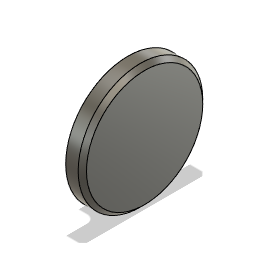
Button Cover Blank v1 (Autodesk Fusion 360 design; units mm, degrees)
Autodesk Fusion 360 part; units mm, degrees
sketch "Sketch1" plane through (0, 0, 0) normal (1, 0, 0) x (0, 0, -1)
  circle A0 centre (0, 0) radius 4
  line L0 (2, 2) -> (-2, 2)
  line L1 (-2, 2) -> (-2, -2)
  line L2 (-2, -2) -> (2, -2)
  line L3 (2, -2) -> (2, 2)
  line L4 (2, 2) -> (-2, -2) construction
  line L5 (-2, 2) -> (2, -2) construction
  dimension "d1" = 8
  dimension "d2" = 4
  dimension "d3" = 4
  constraint coincident A0.centre origin
  constraint horizontal L0
  constraint perpendicular L0 L1
  constraint parallel L0 L2
  constraint parallel L1 L3
  constraint coincident L4 A0.centre
  constraint coincident L5 A0.centre
  measures "d1" diameter of A0
  measures "d2" distance of L0.start L0.end
  measures "d3" distance of L0.start L2.end
extrude "Extrude1" add sketch "Sketch1" along normal blind 2
sketch "Sketch2" plane through (2, 0, 0) normal (1, 0, 0) x (0, 0, -1)
  line L0 (2, 2) -> (2, -2)
  line L1 (2, -2) -> (-2, -2)
  line L2 (-2, -2) -> (-2, 2)
  line L3 (-2, 2) -> (2, 2)
  circle A0 centre (0, 0) radius 4
  circle A1 centre (0, 0) radius 7.5
  dimension "d6" = 15
  constraint coincident A0.centre A1.centre
  measures "d6" diameter of A1
extrude "Extrude2" add sketch "Sketch2" along normal blind 2 contours L0 L1 L2 L3 | A0 | A1
fillet "Fillet1" radius 1 1 edges at (2, -1.4465, 3.7293)
chamfer "Chamfer1" distance 0.5 angle 45 1 edges at (4, -2.7121, 6.9925)
